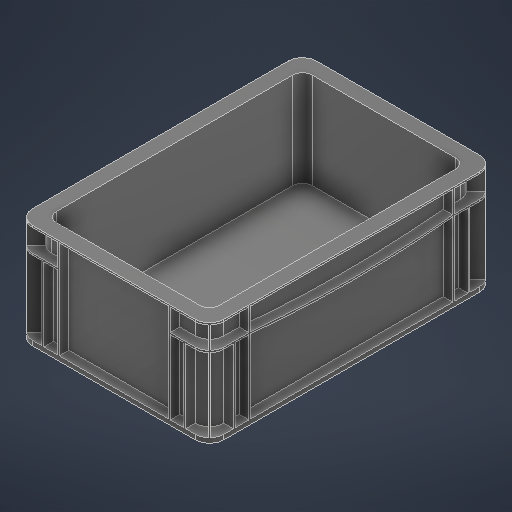
# Autodesk Inventor part: Zeichnung Box
Saved by Autodesk Inventor 2026.2 (Build 302298000, 298)
## iProperties
Created: 2025-11-27
Part Number: Zeichnung Box
Material: Acetalharz, Schwarz
Document SubType Name: Sheet Metal
Designer: Schally
Density: 1.425 g/cm^3
Sheet Metal Rule: Standard_mm
Appearance: Glatt - Schwarz
Author: Schally
Autodesk Inventor part; units mm, degrees
ref_plane "YZ Plane" through (0, 0, 0) normal (1, 0, 0) x (0, 1, 0)
ref_plane "XZ Plane" through (0, 0, 0) normal (0, 1, 0) x (-1, 0, 0)
ref_plane "XY Plane" through (0, 0, 0) normal (0, 0, 1) x (1, 0, 0)
sketch "Skizze1" plane through (0, 0, 0) normal (0, 0, 1) x (1, 0, 0)
  line L0 (-75, 133.5) -> (75, 133.5)
  line L1 (85, 123.5) -> (85, -123.5)
  line L2 (75, -133.5) -> (-75, -133.5)
  line L3 (-85, -123.5) -> (-85, 123.5)
  line L4 (0, -189.7995) -> (0, 189.7995) projected
  line L5 (-122.3137, 0) -> (124.3848, 0) projected
  arc A0 (85, 123.5) -> (75, 133.5) centre (75, 123.5) ccw
  line L6 (75, 133.5) -> (85, 123.5) construction
  line L7 (75, 133.5) -> (89.1421, 133.5) construction
  arc A1 (-75, 133.5) -> (-85, 123.5) centre (-75, 123.5) ccw
  arc A2 (-85, -123.5) -> (-75, -133.5) centre (-75, -123.5) ccw
  arc A3 (75, -133.5) -> (85, -123.5) centre (75, -123.5) ccw
  point P0 (0, 0)
  dimension "d0" = 267
  dimension "d1" = 170
  dimension "d2" = 45
  dimension "d3" = 10
  dimension "d4" = 10
  dimension "d9" = 20
  dimension "d10" = 10
  dimension "d11" = 10
  dimension "d12" = 20
  dimension "d13" = 10
  dimension "d14" = 10
  dimension "d19" = 20
  dimension "d20" = 10
  dimension "d21" = 10
  constraints: 12 end point, 8 point on circle, 4 centre point, 2 horizontal, 2 parallel, 1 equal length, 1 perpendicular, 2 other
  measures "d0" distance between parallel lines of L2 L0
  measures "d1" distance between parallel lines of L3 L1
  measures "d2" angle of L6 L7
  measures "d3" radius of A0
  measures "d4" distance from line of A0.centre L0
  measures "d9" diameter of A1
  measures "d10" distance from line of A1.centre L0
  measures "d11" distance from line of L3 A1.centre
  measures "d12" diameter of A2
  measures "d13" distance from line of L3 A2.centre
  measures "d14" distance from line of L2 A2.centre
  measures "d19" diameter of A3
  measures "d20" distance from line of L2 A3.centre
  measures "d21" distance from line of A3.centre L1
extrude "Extrusion1" add sketch "Skizze1" along normal blind 10
sketch "Skizze2" plane through (0, 0, 10) normal (0, 0, 1) x (1, 0, 0)
  line L0 (75, 133.5) -> (-75, 133.5) projected
  line L1 (75, 133.5) -> (-75, 133.5) projected
  line L2 (75, 133.5) -> (-75, 133.5) projected
  line L3 (75, 133.5) -> (-75, 133.5) projected
  arc A0 (85, 123.5) -> (75, 133.5) centre (75, 123.5) ccw projected
  arc A1 (85, 123.5) -> (75, 133.5) centre (75, 123.5) ccw projected
  arc A2 (85, 123.5) -> (75, 133.5) centre (75, 123.5) ccw projected
  arc A3 (85, 123.5) -> (75, 133.5) centre (75, 123.5) ccw projected
  line L4 (-85, 123.5) -> (-85, -123.5) projected
  line L5 (-85, 123.5) -> (-85, -123.5) projected
  line L6 (-85, 123.5) -> (-85, -123.5) projected
  line L7 (-85, 123.5) -> (-85, -123.5) projected
  arc A4 (-85, -123.5) -> (-75, -133.5) centre (-75, -123.5) ccw projected
  arc A5 (-85, -123.5) -> (-75, -133.5) centre (-75, -123.5) ccw projected
  arc A6 (-85, -123.5) -> (-75, -133.5) centre (-75, -123.5) ccw projected
  arc A7 (-85, -123.5) -> (-75, -133.5) centre (-75, -123.5) ccw projected
  line L8 (85, -123.5) -> (85, 123.5) projected
  line L9 (85, -123.5) -> (85, 123.5) projected
  line L10 (85, -123.5) -> (85, 123.5) projected
  line L11 (85, -123.5) -> (85, 123.5) projected
  line L12 (-75, -133.5) -> (75, -133.5) projected
  line L13 (-75, -133.5) -> (75, -133.5) projected
  line L14 (-75, -133.5) -> (75, -133.5) projected
  line L15 (-75, -133.5) -> (75, -133.5) projected
  line L16 (75, 133.5) -> (-75, 133.5) projected
  arc A8 (85, 123.5) -> (75, 133.5) centre (75, 123.5) ccw projected
  line L17 (85, -123.5) -> (85, 123.5) projected
  arc A9 (75, -133.5) -> (85, -123.5) centre (75, -123.5) ccw projected
  line L18 (-75, -133.5) -> (75, -133.5) projected
  arc A10 (-85, -123.5) -> (-75, -133.5) centre (-75, -123.5) ccw projected
  line L19 (-85, 123.5) -> (-85, -123.5) projected
  arc A11 (-75, 133.5) -> (-85, 123.5) centre (-75, 123.5) ccw projected
  arc A12 (75, -133.5) -> (85, -123.5) centre (75, -123.5) ccw projected
  arc A13 (75, -133.5) -> (85, -123.5) centre (75, -123.5) ccw projected
  arc A14 (75, -133.5) -> (85, -123.5) centre (75, -123.5) ccw projected
  arc A15 (75, -133.5) -> (85, -123.5) centre (75, -123.5) ccw projected
  line L20 (75, 133.5) -> (-75, 133.5) projected
  arc A16 (-75, 133.5) -> (-85, 123.5) centre (-75, 123.5) ccw projected
  line L21 (-85, 123.5) -> (-85, -123.5) projected
  arc A17 (-85, -123.5) -> (-75, -133.5) centre (-75, -123.5) ccw projected
  line L22 (-75, -133.5) -> (75, -133.5) projected
  arc A18 (75, -133.5) -> (85, -123.5) centre (75, -123.5) ccw projected
  line L23 (85, -123.5) -> (85, 123.5) projected
  arc A19 (85, 123.5) -> (75, 133.5) centre (75, 123.5) ccw projected
  arc A20 (-75, 133.5) -> (-85, 123.5) centre (-75, 123.5) ccw projected
  arc A21 (-75, 133.5) -> (-85, 123.5) centre (-75, 123.5) ccw projected
  arc A22 (-75, 133.5) -> (-85, 123.5) centre (-75, 123.5) ccw projected
  arc A23 (-75, 133.5) -> (-85, 123.5) centre (-75, 123.5) ccw projected
  line L24 (-130.3492, 0) -> (130.3492, 0) projected
  line L25 (0, -198.2492) -> (0, 198.2492) projected
  line L26 (90, -123.5) -> (90, 123.5)
  arc A24 (90, 123.5) -> (75, 138.5) centre (75, 123.5) ccw
  line L27 (75, 138.5) -> (-75, 138.5)
  arc A25 (-75, 138.5) -> (-90, 123.5) centre (-75, 123.5) ccw
  line L28 (-90, 123.5) -> (-90, -123.5)
  arc A26 (-90, -123.5) -> (-75, -138.5) centre (-75, -123.5) ccw
  line L29 (-75, -138.5) -> (75, -138.5)
  arc A27 (75, -138.5) -> (90, -123.5) centre (75, -123.5) ccw
  point P0 (0, 0)
  dimension "d25" = 5
  constraints: 8 end point, 8 point on circle, 4 centre point, 10 other
  measures "d25" radial gap between concentric circles of A9 A27
extrude "Extrusion2" add sketch "Skizze2" along normal blind 109
sketch "Skizze3" plane through (0, 0, 119) normal (0, 0, 1) x (1, 0, 0)
  line L0 (-75, -138.5) -> (75, -138.5) projected
  arc A0 (75, -138.5) -> (90, -123.5) centre (75, -123.5) ccw projected
  line L1 (-75, -133.5) -> (75, -133.5) projected
  arc A1 (-85, -123.5) -> (-75, -133.5) centre (-75, -123.5) ccw projected
  arc A2 (-85, -123.5) -> (-75, -133.5) centre (-75, -123.5) ccw projected
  arc A3 (-85, -123.5) -> (-75, -133.5) centre (-75, -123.5) ccw projected
  arc A4 (-90, -123.5) -> (-75, -138.5) centre (-75, -123.5) ccw projected
  line L2 (-75, -138.5) -> (75, -138.5) projected
  line L3 (-75, -138.5) -> (75, -138.5) projected
  line L4 (-75, -138.5) -> (75, -138.5) projected
  line L5 (-75, -133.5) -> (75, -133.5) projected
  line L6 (-75, -133.5) -> (75, -133.5) projected
  line L7 (-75, -133.5) -> (75, -133.5) projected
  arc A5 (75, -133.5) -> (85, -123.5) centre (75, -123.5) ccw projected
  arc A6 (75, -138.5) -> (90, -123.5) centre (75, -123.5) ccw projected
  arc A7 (75, -138.5) -> (90, -123.5) centre (75, -123.5) ccw projected
  arc A8 (-90, -123.5) -> (-75, -138.5) centre (-75, -123.5) ccw projected
  arc A9 (-90, -123.5) -> (-75, -138.5) centre (-75, -123.5) ccw projected
  arc A10 (75, -133.5) -> (85, -123.5) centre (75, -123.5) ccw projected
  arc A11 (75, -133.5) -> (85, -123.5) centre (75, -123.5) ccw projected
  arc A12 (75, -133.5) -> (85, -123.5) centre (75, -123.5) ccw projected
  line L8 (90, -123.5) -> (90, 123.5) projected
  line L9 (85, -123.5) -> (85, 123.5) projected
  line L10 (90, -123.5) -> (90, 123.5) projected
  line L11 (90, -123.5) -> (90, 123.5) projected
  line L12 (90, -123.5) -> (90, 123.5) projected
  line L13 (85, -123.5) -> (85, 123.5) projected
  line L14 (85, -123.5) -> (85, 123.5) projected
  arc A13 (-75, 138.5) -> (-90, 123.5) centre (-75, 123.5) ccw projected
  line L15 (-90, 123.5) -> (-90, -123.5) projected
  arc A14 (-90, -123.5) -> (-75, -138.5) centre (-75, -123.5) ccw projected
  line L16 (-75, -138.5) -> (75, -138.5) projected
  arc A15 (75, -138.5) -> (90, -123.5) centre (75, -123.5) ccw projected
  line L17 (90, -123.5) -> (90, 123.5) projected
  arc A16 (90, 123.5) -> (75, 138.5) centre (75, 123.5) ccw projected
  line L18 (75, 138.5) -> (-75, 138.5) projected
  arc A17 (-75, 138.5) -> (-90, 123.5) centre (-75, 123.5) ccw projected
  line L19 (75, 138.5) -> (-75, 138.5) projected
  arc A18 (90, 123.5) -> (75, 138.5) centre (75, 123.5) ccw projected
  line L20 (90, -123.5) -> (90, 123.5) projected
  arc A19 (75, -138.5) -> (90, -123.5) centre (75, -123.5) ccw projected
  line L21 (-75, -138.5) -> (75, -138.5) projected
  arc A20 (-90, -123.5) -> (-75, -138.5) centre (-75, -123.5) ccw projected
  line L22 (-90, 123.5) -> (-90, -123.5) projected
  arc A21 (85, 123.5) -> (75, 133.5) centre (75, 123.5) ccw projected
  line L23 (75, 133.5) -> (-75, 133.5) projected
  arc A22 (-75, 133.5) -> (-85, 123.5) centre (-75, 123.5) ccw projected
  line L24 (-85, 123.5) -> (-85, -123.5) projected
  arc A23 (-85, -123.5) -> (-75, -133.5) centre (-75, -123.5) ccw projected
  line L25 (-75, -133.5) -> (75, -133.5) projected
  arc A24 (75, -133.5) -> (85, -123.5) centre (75, -123.5) ccw projected
  line L26 (85, -123.5) -> (85, 123.5) projected
  line L27 (75, 133.5) -> (-75, 133.5) projected
  arc A25 (85, 123.5) -> (75, 133.5) centre (75, 123.5) ccw projected
  line L28 (85, -123.5) -> (85, 123.5) projected
  arc A26 (75, -133.5) -> (85, -123.5) centre (75, -123.5) ccw projected
  line L29 (-75, -133.5) -> (75, -133.5) projected
  arc A27 (-85, -123.5) -> (-75, -133.5) centre (-75, -123.5) ccw projected
  line L30 (-85, 123.5) -> (-85, -123.5) projected
  arc A28 (-75, 133.5) -> (-85, 123.5) centre (-75, 123.5) ccw projected
  line L31 (75, 133.5) -> (-75, 133.5) projected
  line L32 (-90, 123.5) -> (-90, -123.5) projected
  line L33 (-85, 123.5) -> (-85, -123.5) projected
  line L34 (-85, 123.5) -> (-85, -123.5) projected
  line L35 (-85, 123.5) -> (-85, -123.5) projected
  line L36 (-85, 123.5) -> (-85, -123.5) projected
  arc A29 (-75, 133.5) -> (-85, 123.5) centre (-75, 123.5) ccw projected
  line L37 (-90, 123.5) -> (-90, -123.5) projected
  line L38 (-90, 123.5) -> (-90, -123.5) projected
  line L39 (-90, 123.5) -> (-90, -123.5) projected
  line L40 (85, -123.5) -> (85, 123.5) projected
  arc A30 (85, 123.5) -> (75, 133.5) centre (75, 123.5) ccw projected
  arc A31 (-75, 138.5) -> (-90, 123.5) centre (-75, 123.5) ccw projected
  arc A32 (90, 123.5) -> (75, 138.5) centre (75, 123.5) ccw projected
  arc A33 (-75, 133.5) -> (-85, 123.5) centre (-75, 123.5) ccw projected
  arc A34 (-75, 133.5) -> (-85, 123.5) centre (-75, 123.5) ccw projected
  arc A35 (-75, 138.5) -> (-90, 123.5) centre (-75, 123.5) ccw projected
  arc A36 (-75, 138.5) -> (-90, 123.5) centre (-75, 123.5) ccw projected
  line L41 (75, 133.5) -> (-75, 133.5) projected
  line L42 (75, 133.5) -> (-75, 133.5) projected
  line L43 (75, 133.5) -> (-75, 133.5) projected
  line L44 (75, 138.5) -> (-75, 138.5) projected
  line L45 (75, 138.5) -> (-75, 138.5) projected
  line L46 (75, 138.5) -> (-75, 138.5) projected
  arc A37 (85, 123.5) -> (75, 133.5) centre (75, 123.5) ccw projected
  arc A38 (85, 123.5) -> (75, 133.5) centre (75, 123.5) ccw projected
  arc A39 (90, 123.5) -> (75, 138.5) centre (75, 123.5) ccw projected
  arc A40 (90, 123.5) -> (75, 138.5) centre (75, 123.5) ccw projected
  arc A41 (90, 123.5) -> (75, 138.5) centre (75, 123.5) ccw projected
  line L47 (75, 138.5) -> (-75, 138.5) projected
  arc A42 (-85, -123.5) -> (-75, -133.5) centre (-75, -123.5) ccw projected
  arc A43 (-90, -123.5) -> (-75, -138.5) centre (-75, -123.5) ccw projected
  arc A44 (75, -138.5) -> (90, -123.5) centre (75, -123.5) ccw projected
  arc A45 (85, 123.5) -> (75, 133.5) centre (75, 123.5) ccw projected
  arc A46 (-75, 133.5) -> (-85, 123.5) centre (-75, 123.5) ccw projected
  arc A47 (-75, 138.5) -> (-90, 123.5) centre (-75, 123.5) ccw projected
  line L48 (-130.3492, 0) -> (130.3492, 0) projected
  line L49 (0, -198.2492) -> (0, 198.2492) projected
  point P0 (0, 0)
  point P1 (-85, -123.5)
  constraints: 9 other
extrude "Extrusion3" cut sketch "Skizze3" against normal blind 100 contours L49 L48 L9 A5 L1 | L1 A1 L24 L48 L49 | L49 L23 A21 L9 L48 | L48 L24 A22 L23 L49
sketch "Skizze4" plane through (0, 0, 10) normal (0, 0, -1) x (-1, 0, 0)
  line L0 (75, -138.5) -> (-75, -138.5) projected
  arc A0 (75, -138.5) -> (90, -123.5) centre (75, -123.5) ccw projected
  arc A1 (90, 123.5) -> (75, 138.5) centre (75, 123.5) ccw projected
  line L1 (-75, 138.5) -> (75, 138.5) projected
  arc A2 (-75, 138.5) -> (-90, 123.5) centre (-75, 123.5) ccw projected
  line L2 (-90, -123.5) -> (-90, 123.5) projected
  arc A3 (-90, -123.5) -> (-75, -138.5) centre (-75, -123.5) ccw projected
  line L3 (75, -138.5) -> (-75, -138.5) projected
  arc A4 (75, -138.5) -> (90, -123.5) centre (75, -123.5) ccw projected
  line L4 (90, 123.5) -> (90, -123.5) projected
  arc A5 (-75, 133.5) -> (-85, 123.5) centre (-75, 123.5) ccw projected
  line L5 (-75, 133.5) -> (75, 133.5) projected
  arc A6 (85, 123.5) -> (75, 133.5) centre (75, 123.5) ccw projected
  line L6 (85, 123.5) -> (85, -123.5) projected
  arc A7 (75, -133.5) -> (85, -123.5) centre (75, -123.5) ccw projected
  line L7 (75, -133.5) -> (-75, -133.5) projected
  arc A8 (-85, -123.5) -> (-75, -133.5) centre (-75, -123.5) ccw projected
  line L8 (-85, -123.5) -> (-85, 123.5) projected
  line L9 (85, -148.5) -> (-85, -148.5)
  line L10 (-100, -133.5) -> (-100, 133.5)
  line L11 (-85, 148.5) -> (85, 148.5)
  line L12 (100, 133.5) -> (100, -133.5)
  arc A9 (100, 133.5) -> (85, 148.5) centre (85, 133.5) ccw
  arc A10 (-85, 148.5) -> (-100, 133.5) centre (-85, 133.5) ccw
  arc A11 (-100, -133.5) -> (-85, -148.5) centre (-85, -133.5) ccw
  arc A12 (85, -148.5) -> (100, -133.5) centre (85, -133.5) ccw
  point P0 (0, 0)
  point P1 (90, -123.5)
  dimension "d68" = 10
  dimension "d69" = 10
  dimension "d70" = 10
  dimension "d71" = 10
  dimension "d73" = 15
  dimension "d74" = 15
  dimension "d75" = 15
  dimension "d76" = 15
  dimension "d77" = 15
  dimension "d78" = 15
  dimension "d79" = 15
  dimension "d80" = 15
  dimension "d81" = 15
  dimension "d82" = 15
  dimension "d83" = 15
  dimension "d84" = 15
  constraints: 8 end point, 8 point on circle, 4 centre point
  measures "d68" distance between parallel lines of L1 L11
  measures "d69" distance between parallel lines of L12 L4
  measures "d70" distance between parallel lines of L9 L0
  measures "d71" distance between parallel lines of L10 L2
  measures "d73" distance from line of L12 L11.end
  measures "d74" distance from line of L11 L12.start
  measures "d75" radius of A9
  measures "d76" horizontal distance of L9.start L12.end
  measures "d77" distance from line of L9.start L12
  measures "d78" distance from line of L10 L9.end
  measures "d79" distance from line of L10.start L9
  measures "d80" distance from line of L10.end L11
  measures "d81" distance from line of L11.start L10
  measures "d82" radius of A10
  measures "d83" radius of A11
  measures "d84" radius of A12
extrude "Extrusion4" add sketch "Skizze4" against normal blind 5 contours L9 A11 L10 A10 L11 A9 L12 A12
sketch "Skizze5" plane through (0, 0, 119) normal (0, 0, 1) x (1, 0, 0)
  line L0 (75, -133.5) -> (-75, -133.5) projected
  arc A0 (-85, -123.5) -> (-75, -133.5) centre (-75, -123.5) ccw projected
  line L1 (-85, -123.5) -> (-85, 123.5) projected
  arc A1 (-75, 133.5) -> (-85, 123.5) centre (-75, 123.5) ccw projected
  line L2 (-75, 133.5) -> (75, 133.5) projected
  arc A2 (85, 123.5) -> (75, 133.5) centre (75, 123.5) ccw projected
  line L3 (85, 123.5) -> (85, -123.5) projected
  arc A3 (75, -133.5) -> (85, -123.5) centre (75, -123.5) ccw projected
  arc A4 (-75, 138.5) -> (-90, 123.5) centre (-75, 123.5) ccw projected
  line L4 (-90, 123.5) -> (-90, -123.5) projected
  arc A5 (-90, -123.5) -> (-75, -138.5) centre (-75, -123.5) ccw projected
  line L5 (-75, -138.5) -> (75, -138.5) projected
  arc A6 (75, -138.5) -> (90, -123.5) centre (75, -123.5) ccw projected
  line L6 (90, -123.5) -> (90, 123.5) projected
  arc A7 (90, 123.5) -> (75, 138.5) centre (75, 123.5) ccw projected
  line L7 (75, 138.5) -> (-75, 138.5) projected
  line L8 (-100, 133.5) -> (-100, -133.5) projected
  arc A8 (-100, -133.5) -> (-85, -148.5) centre (-85, -133.5) ccw projected
  line L9 (-85, -148.5) -> (85, -148.5) projected
  arc A9 (85, -148.5) -> (100, -133.5) centre (85, -133.5) ccw projected
  line L10 (100, -133.5) -> (100, 133.5) projected
  arc A10 (100, 133.5) -> (85, 148.5) centre (85, 133.5) ccw projected
  line L11 (85, 148.5) -> (-85, 148.5) projected
  arc A11 (-85, 148.5) -> (-100, 133.5) centre (-85, 133.5) ccw projected
  line L12 (-90, 123.5) -> (-90, -123.5) projected
  arc A12 (-75, 138.5) -> (-90, 123.5) centre (-75, 123.5) ccw projected
  line L13 (75, 138.5) -> (-75, 138.5) projected
  arc A13 (90, 123.5) -> (75, 138.5) centre (75, 123.5) ccw projected
  line L14 (90, -123.5) -> (90, 123.5) projected
  arc A14 (75, -138.5) -> (90, -123.5) centre (75, -123.5) ccw projected
  line L15 (-75, -138.5) -> (75, -138.5) projected
  arc A15 (-90, -123.5) -> (-75, -138.5) centre (-75, -123.5) ccw projected
  point P0 (0, 0)
extrude "Extrusion5" add sketch "Skizze5" against normal blind 2 contours A11 L11 A10 L10 A9 L9 A8 L8
sketch "Skizze6" plane through (0, 0, 15) normal (0, 0, 1) x (1, 0, 0)
  arc A0 (-75, 133.5) -> (-85, 123.5) centre (-75, 123.5) ccw projected
  arc A1 (-75, 138.5) -> (-90, 123.5) centre (-75, 123.5) ccw construction
  arc A2 (-75, 133.5) -> (-85, 123.5) centre (-75, 123.5) ccw projected
  line L0 (-85, -148.5) -> (85, -148.5) projected
  line L1 (100, -133.5) -> (100, 133.5) projected
  line L2 (85, 148.5) -> (-85, 148.5) projected
  line L3 (-100, 133.5) -> (-100, -133.5) projected
  line L4 (-90, 123.5) -> (-90, -123.5) projected
  arc A3 (-75, 138.5) -> (-90, 123.5) centre (-75, 123.5) ccw projected
  line L5 (75, 138.5) -> (-75, 138.5) projected
  arc A4 (90, 123.5) -> (75, 138.5) centre (75, 123.5) ccw projected
  line L6 (90, -123.5) -> (90, 123.5) projected
  arc A5 (75, -138.5) -> (90, -123.5) centre (75, -123.5) ccw projected
  line L7 (-75, -138.5) -> (75, -138.5) projected
  arc A6 (-90, -123.5) -> (-75, -138.5) centre (-75, -123.5) ccw projected
  line L8 (-100, 107.5) -> (-90, 107.5)
  line L9 (-100, 105.5) -> (-90, 105.5)
  line L10 (-59, 148.5) -> (-59, 138.5)
  line L11 (-57, 148.5) -> (-57, 138.5)
  line L12 (0, -212.6635) -> (0, 214.7345) projected
  line L13 (-146.8345, 0) -> (144.7635, 0) projected
  arc A7 (90, 123.5) -> (75, 138.5) centre (75, 123.5) ccw projected
  line L14 (59, 138.5) -> (59, 148.5)
  line L15 (90, 107.5) -> (100, 107.5)
  line L16 (57, 138.5) -> (57, 148.5)
  line L17 (90, 105.5) -> (100, 105.5)
  line L18 (-75, -138.5) -> (75, -138.5) projected
  line L19 (59, -138.5) -> (59, -148.5)
  line L20 (90, -107.5) -> (100, -107.5)
  line L21 (57, -138.5) -> (57, -148.5)
  line L22 (90, -105.5) -> (100, -105.5)
  line L23 (-59, -148.5) -> (-59, -138.5)
  line L24 (-100, -107.5) -> (-90, -107.5)
  line L25 (-100, -105.5) -> (-90, -105.5)
  line L26 (-57, -148.5) -> (-57, -138.5)
  line L27 (-100, -105.5) -> (-100, -107.5)
  line L28 (-90, -105.5) -> (-90, -107.5)
  arc A8 (-100, -133.5) -> (-85, -148.5) centre (-85, -133.5) ccw projected
  arc A9 (85, -148.5) -> (100, -133.5) centre (85, -133.5) ccw projected
  arc A10 (100, 133.5) -> (85, 148.5) centre (85, 133.5) ccw projected
  arc A11 (-85, 148.5) -> (-100, 133.5) centre (-85, 133.5) ccw projected
  arc A12 (-75, 133.5) -> (-85, 123.5) centre (-75, 123.5) ccw projected
  line L29 (-95.6066, 144.1066) -> (-75, 123.5)
  line L30 (-96.3137, 143.3995) -> (-75.7071, 122.7929)
  line L31 (-94.8995, 144.8137) -> (-74.2929, 124.2071)
  arc A13 (85, 123.5) -> (75, 133.5) centre (75, 123.5) ccw projected
  line L32 (95.6066, 144.1066) -> (75, 123.5)
  line L33 (94.8995, 144.8137) -> (74.2929, 124.2071)
  line L34 (96.3137, 143.3995) -> (75.7071, 122.7929)
  arc A14 (-85, -123.5) -> (-75, -133.5) centre (-75, -123.5) ccw projected
  line L35 (-95.6066, -144.1066) -> (-75, -123.5)
  line L36 (-94.8995, -144.8137) -> (-74.2929, -124.2071)
  line L37 (-96.3137, -143.3995) -> (-75.7071, -122.7929)
  arc A15 (75, -133.5) -> (85, -123.5) centre (75, -123.5) ccw projected
  arc A16 (75, -133.5) -> (85, -123.5) centre (75, -123.5) ccw projected
  line L38 (95.6066, -144.1066) -> (75, -123.5)
  line L39 (96.3137, -143.3995) -> (75.7071, -122.7929)
  line L40 (94.8995, -144.8137) -> (74.2929, -124.2071)
  point P0 (0, 0)
  point P1 (86.2901, 133.3759)
  point P2 (96.2901, 143.3759)
  point P3 (94.8759, 144.7901)
  point P4 (84.8759, 134.7901)
  point P5 (-84.8759, 134.7901)
  point P6 (-94.8759, 144.7901)
  point P7 (-96.2901, 143.3759)
  point P8 (-86.2901, 133.3759)
  point P9 (-94.8759, -144.7901)
  point P10 (-84.8759, -134.7901)
  point P11 (-86.2901, -133.3759)
  point P12 (-96.2901, -143.3759)
  point P13 (96.2901, -143.3759)
  point P14 (86.2901, -133.3759)
  point P15 (84.8759, -134.7901)
  point P16 (94.8759, -144.7901)
  dimension "d41" = 41
  dimension "d42" = 2
  dimension "d43" = 41
  dimension "d44" = 2
  dimension "d45" = 41
  dimension "d46" = 41
  dimension "d47" = 2
  dimension "d48" = 2
  dimension "d51" = 41
  dimension "d52" = 41
  dimension "d53" = 2
  dimension "d54" = 2
  dimension "d57" = 41
  dimension "d58" = 41
  dimension "d61" = 2
  dimension "d62" = 2
  dimension "d85" = 1
  dimension "d86" = 1
  dimension "d87" = 1
  dimension "d88" = 1
  dimension "d89" = 1
  dimension "d90" = 1
  dimension "d91" = 1
  dimension "d92" = 1
  constraints: 60 end point, 16 parallel, 15 point on line, 8 perpendicular, 4 point on circle, 2 collinear
  measures "d41" distance between parallel lines of L8 L2
  measures "d42" distance between parallel lines of L8 L9
  measures "d43" distance between parallel lines of L3 L10
  measures "d44" distance between parallel lines of L10 L11
  measures "d45" distance between parallel lines of L1 L14
  measures "d46" distance between parallel lines of L15 L2
  measures "d47" distance between parallel lines of L14 L16
  measures "d48" distance between parallel lines of L15 L17
  measures "d51" distance between parallel lines of L19 L1
  measures "d52" distance between parallel lines of L20 L0
  measures "d53" distance between parallel lines of L19 L21
  measures "d54" distance between parallel lines of L20 L22
  measures "d57" distance between parallel lines of L3 L23
  measures "d58" distance between parallel lines of L24 L0
  measures "d61" distance between parallel lines of L24 L25
  measures "d62" distance between parallel lines of L23 L26
  measures "d85" distance between parallel lines of L29 L30
  measures "d86" distance between parallel lines of L29 L31
  measures "d87" distance between parallel lines of L32 L33
  measures "d88" distance between parallel lines of L32 L34
  measures "d89" distance between parallel lines of L35 L36
  measures "d90" distance between parallel lines of L35 L37
  measures "d91" distance between parallel lines of L38 L39
  measures "d92" distance between parallel lines of L38 L40
extrude "Extrusion6" add sketch "Skizze6" along normal blind 103 contours A3 L29 A11 L31 | A3 L30 A11 L29 | L10 L2 L11 L5 | L4 L9 L3 L8 | L16 L2 L14 L5 | L4 L24 L3 L25 | L26 L0 L23 L7 | L7 L19 L0 L21 | L22 L1 L20 L6 | L6 L15 L1 L17 | L33 A10 L32 A4 | L32 A10 L34 A4 | A6 L35 A8 L37 | L36 A8 L35 A6 | A5 L38 A9 L40 | L39 A9 L38 A5
sketch "Skizze8" plane through (0, 0, 15) normal (0, 0, 1) x (1, 0, 0)
  arc A0 (-100, -133.5) -> (-85, -148.5) centre (-85, -133.5) ccw projected
  line L0 (-85, -148.5) -> (85, -148.5) projected
  arc A1 (85, -148.5) -> (100, -133.5) centre (85, -133.5) ccw projected
  line L1 (100, -133.5) -> (100, 133.5) projected
  arc A2 (100, 133.5) -> (85, 148.5) centre (85, 133.5) ccw projected
  line L2 (85, 148.5) -> (-85, 148.5) projected
  arc A3 (-85, 148.5) -> (-100, 133.5) centre (-85, 133.5) ccw projected
  line L3 (-100, 133.5) -> (-100, -133.5) projected
  line L4 (75, -133.5) -> (-75, -133.5) projected
  arc A4 (-85, -123.5) -> (-75, -133.5) centre (-75, -123.5) ccw projected
  line L5 (-85, -123.5) -> (-85, 123.5) projected
  arc A5 (-75, 133.5) -> (-85, 123.5) centre (-75, 123.5) ccw projected
  line L6 (-75, 133.5) -> (75, 133.5) projected
  arc A6 (85, 123.5) -> (75, 133.5) centre (75, 123.5) ccw projected
  line L7 (85, 123.5) -> (85, -123.5) projected
  arc A7 (75, -133.5) -> (85, -123.5) centre (75, -123.5) ccw projected
  line L8 (75, 148.5) -> (75, 138.5)
  line L9 (75, 138.5) -> (59, 138.5) projected
  line L10 (73, 148.5) -> (73, 138.5)
  line L11 (90, 123.5) -> (100, 123.5)
  line L12 (90, 121.5) -> (100, 121.5)
  line L13 (-75, 138.5) -> (-75, 148.5)
  line L14 (-85, 148.5) -> (85, 148.5) projected
  line L15 (-73, 138.5) -> (-73, 148.5)
  line L16 (-90, 123.5) -> (-100, 123.5)
  line L17 (-90, 121.5) -> (-100, 121.5)
  line L18 (-90, -123.5) -> (-100, -123.5)
  line L19 (-90, -121.5) -> (-100, -121.5)
  line L20 (-75, -138.5) -> (-75, -148.5)
  line L21 (-73, -138.5) -> (-73, -148.5)
  arc A8 (75, -138.5) -> (84.8759, -134.7901) centre (75, -123.5) ccw projected
  line L22 (75, -138.5) -> (75, -148.5)
  line L23 (59, -148.5) -> (85, -148.5) projected
  line L24 (73, -148.5) -> (73, -136.3452)
  arc A9 (73, -136.3452) -> (83.5591, -133.2848) centre (75, -123.5) ccw
  arc A10 (86.2901, -133.3759) -> (90, -123.5) centre (75, -123.5) ccw projected
  line L25 (90, -123.5) -> (100, -123.5)
  line L26 (100, -121.5) -> (87.8452, -121.5)
  arc A11 (84.7848, -132.0591) -> (87.8452, -121.5) centre (75, -123.5) ccw
  line L27 (-75, -138.5) -> (-59, -138.5) projected
  arc A12 (-84.8759, -134.7901) -> (-75, -138.5) centre (-75, -123.5) ccw projected
  line L28 (-57, -138.5) -> (57, -138.5) projected
  line L29 (-85, -123.5) -> (-85, 123.5) projected
  line L30 (-90, -105.5) -> (-90, 105.5) projected
  line L31 (-90, 105.5) -> (-90, -105.5) projected
  line L32 (-90, -107.5) -> (-90, -123.5) projected
  line L33 (-90, -123.5) -> (-90, -107.5) projected
  arc A13 (-90, -123.5) -> (-86.2901, -133.3759) centre (-75, -123.5) ccw projected
  arc A14 (-90, -123.5) -> (-86.2901, -133.3759) centre (-75, -123.5) ccw projected
  arc A15 (-84.8759, -134.7901) -> (-75, -138.5) centre (-75, -123.5) ccw projected
  arc A16 (-84.8759, -134.7901) -> (-75, -138.5) centre (-75, -123.5) ccw projected
  line L34 (-59, -138.5) -> (-75, -138.5) projected
  line L35 (-75, -138.5) -> (-59, -138.5) projected
  line L36 (-57, -138.5) -> (57, -138.5) projected
  line L37 (57, -138.5) -> (-57, -138.5) projected
  line L38 (59, -138.5) -> (75, -138.5) projected
  line L39 (75, -138.5) -> (59, -138.5) projected
  arc A17 (75, -138.5) -> (84.8759, -134.7901) centre (75, -123.5) ccw projected
  arc A18 (75, -138.5) -> (84.8759, -134.7901) centre (75, -123.5) ccw projected
  arc A19 (86.2901, -133.3759) -> (90, -123.5) centre (75, -123.5) ccw projected
  arc A20 (86.2901, -133.3759) -> (90, -123.5) centre (75, -123.5) ccw projected
  line L40 (90, -107.5) -> (90, -123.5) projected
  line L41 (90, -123.5) -> (90, -107.5) projected
  line L42 (90, 105.5) -> (90, -105.5) projected
  line L43 (90, -105.5) -> (90, 105.5) projected
  line L44 (-90, 107.5) -> (-90, 123.5) projected
  line L45 (-90, 123.5) -> (-90, 107.5) projected
  arc A21 (-86.2901, 133.3759) -> (-90, 123.5) centre (-75, 123.5) ccw projected
  arc A22 (-86.2901, 133.3759) -> (-90, 123.5) centre (-75, 123.5) ccw projected
  arc A23 (-75, 138.5) -> (-84.8759, 134.7901) centre (-75, 123.5) ccw projected
  arc A24 (-75, 138.5) -> (-84.8759, 134.7901) centre (-75, 123.5) ccw projected
  line L46 (-59, 138.5) -> (-75, 138.5) projected
  line L47 (-75, 138.5) -> (-59, 138.5) projected
  line L48 (-57, 138.5) -> (57, 138.5) projected
  line L49 (57, 138.5) -> (-57, 138.5) projected
  arc A25 (84.8759, 134.7901) -> (75, 138.5) centre (75, 123.5) ccw projected
  arc A26 (84.8759, 134.7901) -> (75, 138.5) centre (75, 123.5) ccw projected
  line L50 (59, 138.5) -> (75, 138.5) projected
  line L51 (75, 138.5) -> (59, 138.5) projected
  arc A27 (90, 123.5) -> (86.2901, 133.3759) centre (75, 123.5) ccw projected
  arc A28 (90, 123.5) -> (86.2901, 133.3759) centre (75, 123.5) ccw projected
  line L52 (90, 107.5) -> (90, 123.5) projected
  line L53 (90, 123.5) -> (90, 107.5) projected
  point P0 (0, 0)
  point P1 (90, -121.5)
  point P2 (73, -138.5)
  dimension "d93" = 25
  dimension "d94" = 2
  dimension "d95" = 2
  dimension "d96" = 25
  dimension "d97" = 2
  dimension "d98" = 2
  dimension "d99" = 25
  dimension "d100" = 2
  dimension "d102" = 2
  dimension "d103" = 2
  dimension "d104" = 2
  constraints: 32 end point, 9 point on line, 6 parallel, 6 perpendicular, 4 point on circle, 2 centre point, 1 horizontal, 1 vertical, 2 other
  measures "d93" distance between parallel lines of L8 L1
  measures "d94" distance between parallel lines of L8 L10
  measures "d95" distance between parallel lines of L11 L12
  measures "d96" distance between parallel lines of L13 L3
  measures "d97" distance between parallel lines of L13 L15
  measures "d98" distance between parallel lines of L16 L17
  measures "d99" distance between parallel lines of L0 L18
  measures "d100" distance between parallel lines of L18 L19
  measures "d102" distance between parallel lines of L20 L21
  measures "d103" distance between parallel lines of L22 L24
  measures "d104" distance between parallel lines of L25 L26
extrude "Extrusion7" add sketch "Skizze8" along normal blind 77 contours L3 L19 L32 L18 | L20 L27 L21 L0 | L3 L16 L44 L17 | L24 L38 L22 L0 | L2 L15 L46 L13 | L25 L40 L26 L1 | L2 L8 L9 L10 | L12 L52 L11 L1
sketch "Skizze9" plane through (0, 0, 92) normal (0, 0, 1) x (1, 0, 0)
  line L0 (-100, 123.5) -> (-90, 123.5) projected
  arc A0 (-86.2901, 133.3759) -> (-90, 123.5) centre (-75, 123.5) ccw projected
  line L1 (-86.2901, 133.3759) -> (-96.2901, 143.3759) projected
  arc A1 (-96.2901, 143.3759) -> (-100, 133.5) centre (-85, 133.5) ccw projected
  line L2 (-100, 133.5) -> (-100, 123.5) projected
  line L3 (-90, 121.5) -> (-100, 121.5) projected
  line L4 (-100, 121.5) -> (-100, 107.5) projected
  line L5 (-100, 107.5) -> (-90, 107.5) projected
  line L6 (-90, 121.5) -> (-90, 107.5) projected
  line L7 (-90, 123.5) -> (-100, 123.5) projected
  line L8 (-100, 123.5) -> (-100, 121.5) projected
  line L9 (-100, 121.5) -> (-90, 121.5) projected
  line L10 (-90, 123.5) -> (-90, 121.5) projected
  line L11 (-73, 138.5) -> (-73, 148.5) projected
  line L12 (-73, 148.5) -> (-75, 148.5) projected
  line L13 (-75, 148.5) -> (-75, 138.5) projected
  line L14 (-73, 138.5) -> (-75, 138.5) projected
  line L15 (-73, 148.5) -> (-73, 138.5) projected
  line L16 (-59, 138.5) -> (-73, 138.5) projected
  line L17 (-59, 138.5) -> (-59, 148.5) projected
  line L18 (-59, 148.5) -> (-73, 148.5) projected
  line L19 (-75, 138.5) -> (-75, 148.5) projected
  line L20 (-75, 148.5) -> (-85, 148.5) projected
  arc A2 (-85, 148.5) -> (-94.8759, 144.7901) centre (-85, 133.5) ccw projected
  line L21 (-94.8759, 144.7901) -> (-84.8759, 134.7901) projected
  arc A3 (-75, 138.5) -> (-84.8759, 134.7901) centre (-75, 123.5) ccw projected
  arc A4 (-85, 148.5) -> (-100, 133.5) centre (-85, 133.5) ccw projected
  arc A5 (-96.2901, 143.3759) -> (-100, 133.5) centre (-85, 133.5) ccw projected
  arc A6 (-96.2901, 143.3759) -> (-100, 133.5) centre (-85, 133.5) ccw projected
  arc A7 (-85, 148.5) -> (-100, 133.5) centre (-85, 133.5) ccw projected
  arc A8 (-85, 148.5) -> (-94.8759, 144.7901) centre (-85, 133.5) ccw projected
  arc A9 (-85, 148.5) -> (-94.8759, 144.7901) centre (-85, 133.5) ccw projected
  line L22 (75, 138.5) -> (73, 138.5) projected
  line L23 (75, 138.5) -> (75, 148.5) projected
  line L24 (75, 148.5) -> (73, 148.5) projected
  line L25 (73, 148.5) -> (73, 138.5) projected
  line L26 (73, 138.5) -> (73, 148.5) projected
  line L27 (73, 148.5) -> (59, 148.5) projected
  line L28 (59, 148.5) -> (59, 138.5) projected
  line L29 (73, 138.5) -> (59, 138.5) projected
  line L30 (75, 148.5) -> (75, 138.5) projected
  arc A10 (84.8759, 134.7901) -> (75, 138.5) centre (75, 123.5) ccw projected
  line L31 (84.8759, 134.7901) -> (94.8759, 144.7901) projected
  arc A11 (94.8759, 144.7901) -> (85, 148.5) centre (85, 133.5) ccw projected
  line L32 (85, 148.5) -> (75, 148.5) projected
  arc A12 (100, 133.5) -> (96.2901, 143.3759) centre (85, 133.5) ccw projected
  arc A13 (100, 133.5) -> (85, 148.5) centre (85, 133.5) ccw projected
  arc A14 (94.8759, 144.7901) -> (85, 148.5) centre (85, 133.5) ccw projected
  arc A15 (94.8759, 144.7901) -> (85, 148.5) centre (85, 133.5) ccw projected
  arc A16 (100, 133.5) -> (85, 148.5) centre (85, 133.5) ccw projected
  arc A17 (100, 133.5) -> (96.2901, 143.3759) centre (85, 133.5) ccw projected
  arc A18 (100, 133.5) -> (96.2901, 143.3759) centre (85, 133.5) ccw projected
  line L33 (90, 123.5) -> (100, 123.5) projected
  line L34 (100, 123.5) -> (100, 133.5) projected
  arc A19 (100, 133.5) -> (96.2901, 143.3759) centre (85, 133.5) ccw projected
  line L35 (96.2901, 143.3759) -> (86.2901, 133.3759) projected
  arc A20 (90, 123.5) -> (86.2901, 133.3759) centre (75, 123.5) ccw projected
  line L36 (100, 121.5) -> (90, 121.5) projected
  line L37 (90, 107.5) -> (90, 121.5) projected
  line L38 (90, 107.5) -> (100, 107.5) projected
  line L39 (100, 107.5) -> (100, 121.5) projected
  line L40 (90, 121.5) -> (100, 121.5) projected
  line L41 (100, 121.5) -> (100, 123.5) projected
  line L42 (100, 123.5) -> (90, 123.5) projected
  line L43 (90, 121.5) -> (90, 123.5) projected
  line L44 (100, -123.5) -> (90, -123.5) projected
  arc A21 (86.2901, -133.3759) -> (90, -123.5) centre (75, -123.5) ccw projected
  line L45 (86.2901, -133.3759) -> (96.2901, -143.3759) projected
  arc A22 (96.2901, -143.3759) -> (100, -133.5) centre (85, -133.5) ccw projected
  line L46 (100, -133.5) -> (100, -123.5) projected
  line L47 (90, -121.5) -> (100, -121.5) projected
  line L48 (100, -121.5) -> (100, -107.5) projected
  line L49 (100, -107.5) -> (90, -107.5) projected
  line L50 (90, -121.5) -> (90, -107.5) projected
  line L51 (90, -123.5) -> (100, -123.5) projected
  line L52 (100, -123.5) -> (100, -121.5) projected
  line L53 (100, -121.5) -> (90, -121.5) projected
  line L54 (90, -123.5) -> (90, -121.5) projected
  line L55 (73, -138.5) -> (73, -148.5) construction
  line L56 (73, -148.5) -> (75, -148.5) construction
  line L57 (75, -148.5) -> (75, -138.5) construction
  line L58 (73, -138.5) -> (75, -138.5) construction
  line L59 (73, -148.5) -> (73, -138.5) construction
  line L60 (59, -138.5) -> (73, -138.5) construction
  line L61 (59, -138.5) -> (59, -148.5) construction
  line L62 (59, -148.5) -> (73, -148.5) construction
  line L63 (75, -138.5) -> (75, -148.5) construction
  line L64 (75, -148.5) -> (85, -148.5) construction
  arc A23 (85, -148.5) -> (94.8759, -144.7901) centre (85, -133.5) ccw construction
  line L65 (94.8759, -144.7901) -> (84.8759, -134.7901) construction
  arc A24 (75, -138.5) -> (84.8759, -134.7901) centre (75, -123.5) ccw construction
  arc A25 (96.2901, -143.3759) -> (100, -133.5) centre (85, -133.5) ccw construction
  arc A26 (85, -148.5) -> (100, -133.5) centre (85, -133.5) ccw construction
  arc A27 (85, -148.5) -> (94.8759, -144.7901) centre (85, -133.5) ccw construction
  arc A28 (85, -148.5) -> (94.8759, -144.7901) centre (85, -133.5) ccw construction
  arc A29 (85, -148.5) -> (100, -133.5) centre (85, -133.5) ccw construction
  arc A30 (96.2901, -143.3759) -> (100, -133.5) centre (85, -133.5) ccw construction
  line L66 (-73, -138.5) -> (-73, -148.5) projected
  line L67 (-73, -148.5) -> (-59, -148.5) projected
  line L68 (-59, -148.5) -> (-59, -138.5) projected
  line L69 (-73, -138.5) -> (-59, -138.5) projected
  line L70 (-75, -138.5) -> (-75, -148.5) projected
  line L71 (-75, -148.5) -> (-73, -148.5) projected
  line L72 (-73, -148.5) -> (-73, -138.5) projected
  line L73 (-75, -138.5) -> (-73, -138.5) projected
  line L74 (-75, -148.5) -> (-75, -138.5) projected
  arc A31 (-84.8759, -134.7901) -> (-75, -138.5) centre (-75, -123.5) ccw projected
  line L75 (-84.8759, -134.7901) -> (-94.8759, -144.7901) projected
  arc A32 (-94.8759, -144.7901) -> (-85, -148.5) centre (-85, -133.5) ccw projected
  line L76 (-85, -148.5) -> (-75, -148.5) projected
  line L77 (-90, -123.5) -> (-100, -123.5) projected
  line L78 (-100, -123.5) -> (-100, -133.5) projected
  arc A33 (-100, -133.5) -> (-96.2901, -143.3759) centre (-85, -133.5) ccw projected
  line L79 (-96.2901, -143.3759) -> (-86.2901, -133.3759) projected
  arc A34 (-90, -123.5) -> (-86.2901, -133.3759) centre (-75, -123.5) ccw projected
  line L80 (-90, -121.5) -> (-100, -121.5) projected
  line L81 (-100, -121.5) -> (-100, -123.5) projected
  line L82 (-100, -123.5) -> (-90, -123.5) projected
  line L83 (-90, -121.5) -> (-90, -123.5) projected
  line L84 (-100, -121.5) -> (-90, -121.5) projected
  line L85 (-90, -107.5) -> (-90, -121.5) projected
  line L86 (-90, -107.5) -> (-100, -107.5) projected
  line L87 (-100, -107.5) -> (-100, -121.5) projected
  arc A35 (-100, -133.5) -> (-85, -148.5) centre (-85, -133.5) ccw projected
  arc A36 (-94.8759, -144.7901) -> (-85, -148.5) centre (-85, -133.5) ccw projected
  arc A37 (-94.8759, -144.7901) -> (-85, -148.5) centre (-85, -133.5) ccw projected
  arc A38 (-100, -133.5) -> (-85, -148.5) centre (-85, -133.5) ccw projected
  arc A39 (-100, -133.5) -> (-96.2901, -143.3759) centre (-85, -133.5) ccw projected
  arc A40 (-100, -133.5) -> (-96.2901, -143.3759) centre (-85, -133.5) ccw projected
  arc A41 (-75, 138.5) -> (-90, 123.5) centre (-75, 123.5) ccw
  line L88 (-90, 123.5) -> (-90, 107.5)
  line L89 (-90, 107.5) -> (-100, 107.5)
  line L90 (-100, 133.5) -> (-100, 107.5)
  arc A42 (-85, 148.5) -> (-100, 133.5) centre (-85, 133.5) ccw
  line L91 (-59, 148.5) -> (-85, 148.5)
  line L92 (-59, 138.5) -> (-75, 138.5)
  line L93 (-59, 138.5) -> (-59, 148.5)
  arc A43 (100, 133.5) -> (85, 148.5) centre (85, 133.5) ccw
  arc A44 (90, 123.5) -> (75, 138.5) centre (75, 123.5) ccw
  line L94 (100, 133.5) -> (100, 107.5)
  line L95 (90, 123.5) -> (90, 107.5)
  line L96 (100, -133.5) -> (100, 133.5) projected
  line L97 (90, 107.5) -> (100, 107.5)
  line L98 (85, 148.5) -> (59, 148.5)
  line L99 (75, 138.5) -> (59, 138.5)
  line L100 (59, 138.5) -> (59, 148.5)
  arc A45 (-90, -123.5) -> (-75, -138.5) centre (-75, -123.5) ccw
  arc A46 (-100, -133.5) -> (-85, -148.5) centre (-85, -133.5) ccw
  line L101 (-90, -123.5) -> (-90, -107.5)
  line L102 (-100, -107.5) -> (-90, -107.5)
  line L103 (-100, -107.5) -> (-100, -133.5)
  line L104 (-75, -138.5) -> (-59, -138.5)
  line L105 (-59, -138.5) -> (-59, -148.5)
  line L106 (-85, -148.5) -> (-59, -148.5)
  arc A47 (85, -148.5) -> (100, -133.5) centre (85, -133.5) ccw
  arc A48 (75, -138.5) -> (90, -123.5) centre (75, -123.5) ccw
  line L107 (90, -123.5) -> (90, -107.5)
  line L108 (90, -107.5) -> (100, -107.5)
  line L109 (100, -107.5) -> (100, -133.5)
  line L110 (59, -138.5) -> (75, -138.5)
  line L111 (59, -138.5) -> (59, -148.5)
  line L112 (59, -148.5) -> (85, -148.5)
  point P0 (0, 0)
  point P1 (96.2901, 143.3759)
  constraints: 48 end point, 32 point on circle, 9 collinear, 8 centre point, 7 concentric, 5 point on line, 5 tangent, 4 perpendicular, 3 horizontal, 3 vertical, 3 other
extrude "Extrusion8" add sketch "Skizze9" along normal blind 2 contours L2 A1 L1 A0 L0 | L0 L10 L3 L8 | L3 L6 L5 L4 | L21 A2 L20 L13 A3 | L13 L12 L11 L14 | L11 L18 L17 L16 | L48 L47 L50 L49 | L22 L25 L24 L23 | L23 L32 A11 L31 A10 | L29 L28 L27 L25 | L35 A12 L34 L33 A20 | L33 L41 L36 L43 | L36 L39 L38 L37 | L52 L44 L54 L47 | L46 A22 L45 A21 L44 | L45 A47 L112 L111 L110 A48 | L69 L68 L67 L66 | L66 L71 L70 L73 | L70 L76 A32 L75 A31 | L75 A35 L79 A45 | L79 A33 L78 L77 A34 | L77 L81 L80 L83 | L80 L87 L86 L85
sketch "Skizze10" plane through (90, -105.5, 117) normal (1, 0, 0) x (0, 0, -1)
  line L0 (25, -16) -> (25, -2) projected
  line L1 (25, -2) -> (25, 0)
  line L2 (102, 0) -> (0, 0) projected
  line L3 (25, 227) -> (25, 213) projected
  line L4 (25, 213) -> (25, 211)
  line L5 (0, 211) -> (102, 211) projected
  line L6 (23, 213) -> (23, 211)
  line L7 (23, -2) -> (23, -28) projected
  line L8 (23, -2) -> (23, 0)
  arc A0 (23, 0) -> (23, 211) centre (-1087.525, 105.5) ccw
  line L9 (25, 213) -> (25, 211.0947)
  arc A1 (25, -0.0947) -> (25, 211.0947) centre (-1087.525, 105.5) ccw
  line L10 (25, -0.0947) -> (25, -2)
  line L11 (25, -2) -> (25, -28)
  line L12 (0, 211) -> (0, 0) projected
  point P0 (117, 105.5)
  point P1 (28, 105.5)
  point P2 (25.009, 0)
  point P3 (25.009, 211)
  dimension "d115" = 2
  dimension "d116" = 28
  constraints: 14 end point, 5 point on circle, 4 point on line, 2 centre point, 2 perpendicular, 2 vertical, 3 other
  measures "d115" radial gap between concentric circles of A0 A1
  measures "d116" distance from line of L12 point (28, 105.5)
extrude "Extrusion9" add sketch "Skizze10" along normal blind 10 contours L2 A0 L5 A1
sketch "Skizze11" plane through (-90, -105.5, 117) normal (-1, 0, 0) x (0, 0, 1)
  line L0 (-23, 0) -> (0, 0) projected
  line L1 (-23, 211) -> (0, 211) projected
  arc A0 (-23, 211) -> (-23, 0) centre (1087.525, 105.5) ccw projected
  line L2 (-23, 213) -> (0, 213) projected
  line L3 (0, 239) -> (0, 213) projected
  line L4 (2, 239) -> (0, 239) projected
  line L5 (2, -28) -> (2, 239) projected
  line L6 (2, -28) -> (0, -28) projected
  line L7 (0, -2) -> (0, -28) projected
  line L8 (-23, -2) -> (0, -2) projected
  line L9 (-23, -28) -> (-23, -2) projected
  line L10 (-25, -28) -> (-23, -28) projected
  line L11 (-25, -28) -> (-25, -18) projected
  line L12 (-102, -18) -> (-25, -18) projected
  line L13 (-102, -28) -> (-102, -18) projected
  line L14 (-107, -28) -> (-102, -28) projected
  line L15 (-107, 239) -> (-107, -28) projected
  line L16 (-107, 239) -> (-102, 239) projected
  line L17 (-102, 229) -> (-102, 239) projected
  line L18 (-102, 229) -> (-25, 229) projected
  line L19 (-25, 229) -> (-25, 239) projected
  line L20 (-25, 239) -> (-23, 239) projected
  line L21 (-23, 213) -> (-23, 239) projected
  line L22 (-102, -2) -> (-25, -2) projected
  line L23 (-102, -16) -> (-102, -2) projected
  line L24 (-102, -16) -> (-25, -16) projected
  line L25 (-25, -16) -> (-25, -2) projected
  line L26 (-102, 0) -> (-102, 211) projected
  line L27 (-25, 213) -> (-25, 227) projected
  line L28 (-102, 227) -> (-25, 227) projected
  line L29 (-102, 213) -> (-102, 227) projected
  line L30 (-102, 213) -> (-25, 213) projected
  line L31 (0, 211) -> (-102, 211) projected
  line L32 (-102, 0) -> (0, 0) projected
  line L33 (0, 211) -> (0, 0) projected
  arc A1 (-25.009, 211) -> (-25.009, 0) centre (1087.525, 105.5) ccw projected
  line L34 (-102, 211) -> (-25.009, 211) projected
  line L35 (-102, 0) -> (-25.009, 0) projected
  point P0 (-117, 105.5)
  point P1 (-25, 0)
  point P2 (-25, 211)
  point P3 (-25.009, 211)
  point P4 (-25.009, 0)
extrude "Extrusion10" add sketch "Skizze11" along normal blind 10 contours L32 A1 L31 A0
equation "\"Biegeradius\" = Stärke"
equation "\"BreiteBiegungsfreistellung\" = Stärke"
equation "\"TiefeBiegungsfreistellung\" = 0.5 * Stärke"
equation "\"GrößeEckenfreistellung\" = 4 * Stärke"
equation "\"MinimalRest\" = 2 * Stärke"
equation "\"Übergangsradius\" = Biegeradius"
equation "\"JacobiRadiusGröße\" = Biegeradius"
equation "\"Abstandsgröße\" = Stärke"
equation "\"Stärke\" = 0.5"
